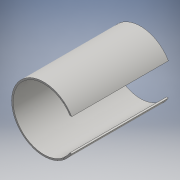
# Autodesk Inventor part: nasel2
Saved by Autodesk Inventor 2016 SP1 (Build 200210100, 210)
## iProperties
Created: 2017-01-27
Part Number: nasel2
Material: 一般
Document SubType Name: Modeling
Designer: p_admin
Density: 1 g/cm^3
Appearance: 既定
Author: p_admin
Autodesk Inventor part; units mm, degrees
ref_plane "YZ Plane" through (0, 0, 0) normal (1, 0, 0) x (0, 1, 0)
ref_plane "XZ Plane" through (0, 0, 0) normal (0, 1, 0) x (-1, 0, 0)
ref_plane "XY Plane" through (0, 0, 0) normal (0, 0, 1) x (1, 0, 0)
sketch "スケッチ1" plane through (0, 0, 0) normal (0, 1, 0) x (-1, 0, 0)
  circle A0 centre (0, 0) radius 190
  circle A1 centre (0, 0) radius 200
  dimension "d0" = 380
  dimension "d1" = 400
  constraints: 2 centre point, 2 coincident
  measures "d0" diameter of A0
  measures "d1" diameter of A1
extrude "押し出し1" add sketch "スケッチ1" along normal blind 600
sketch "スケッチ2" plane through (0, 600, 0) normal (0, 1, 0) x (1, 0, 0)
  line L0 (129.7402, -100) -> (207.3089, -100)
  line L1 (207.3089, -100) -> (207.3089, 100)
  line L2 (207.3089, 100) -> (129.7402, 100)
  line L3 (129.7402, 100) -> (129.7402, -100)
  line L4 (129.7402, -100) -> (207.3089, 100) construction
  line L5 (207.3089, -100) -> (129.7402, 100) construction
  circle A0 centre (0, 0) radius 200 projected
  line L6 (122, -150) -> (128, -150)
  line L7 (128, -150) -> (128, 150)
  line L8 (128, 150) -> (122, 150)
  line L9 (122, 150) -> (122, -150)
  line L10 (122, -150) -> (128, 150) construction
  line L11 (128, -150) -> (122, 150) construction
  point P0 (168.5246, 0)
  point P1 (125, 0)
  dimension "d4" = 200
  dimension "d5" = 125
  dimension "d6" = 6
  dimension "d7" = 300
  constraints: 24 end point, 4 midpoint, 4 parallel, 2 horizontal, 2 perpendicular
  measures "d4" distance of L1.end L0.end
  measures "d5" distance of point (125, 0) A0.centre
  measures "d6" distance of L8.end L7.end
  measures "d7" distance of L7.end L6.end
extrude "押し出し2" cut sketch "スケッチ2" against normal blind 706.25 contours L3 L2 A0 L0 | A0 L2 L1 L0 | L9 L8 L7 L6 picked at (153.1601, 0)
